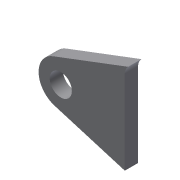
# Autodesk Inventor part: Soporte pivote freno
Saved by Autodesk Inventor 2019 (Build 230136000, 136)
## iProperties
Created: 2020-02-07
Part Number: Soporte pivote freno
Material: Generic
Document SubType Name: Modeling
Designer: Juan Carlos Botero
Density: 1 g/cm^3
Appearance: Default
Author: Juan Carlos Botero
Autodesk Inventor part; units mm, degrees
ref_plane "YZ Plane" through (0, 0, 0) normal (1, 0, 0) x (0, 1, 0)
ref_plane "XZ Plane" through (0, 0, 0) normal (0, 1, 0) x (-1, 0, 0)
ref_plane "XY Plane" through (0, 0, 0) normal (0, 0, 1) x (1, 0, 0)
sketch "Sketch1" plane through (0, 0, 0) normal (0, 0, 1) x (1, 0, 0)
  circle A0 centre (17.6912, 0) radius 5
  circle A1 centre (17.6912, 0) radius 10
  line L0 (17.2789, 9.9915) -> (48.052, 11.2613)
  ellipse E0 centre (55.5218, 7.7366) end of major axis (46.5416, 7.7366) minor radius 6.35 (55.5218, 14.0866) -> (46.5416, 7.7366) ccw
  line L1 (55.5218, 14.0866) -> (108.272, 14.0866)
  ellipse E1 centre (108.272, 7.7366) end of major axis (99.2917, 7.7366) minor radius 6.35 (117.2522, 7.7366) -> (108.272, 14.0866) ccw
  line L2 (117.2522, 7.7366) -> (117.2522, -29.5634)
  ellipse E2 centre (108.272, -29.5634) end of major axis (99.2917, -29.5634) minor radius 6.35 (108.272, -35.9134) -> (117.2522, -29.5634) ccw
  line L3 (108.272, -35.9134) -> (55.5218, -35.9134)
  ellipse E3 centre (55.5218, -29.5634) end of major axis (46.5416, -29.5634) minor radius 6.35 (46.5416, -29.5634) -> (55.5218, -35.9134) ccw
  line L4 (46.5416, -29.5634) -> (46.5416, 7.7366)
  line L5 (108.272, 10.9116) -> (55.5218, 10.9116)
  ellipse E4 centre (55.5218, 7.7366) end of major axis (51.0317, 7.7366) minor radius 3.175 (55.5218, 10.9116) -> (51.0317, 7.7366) ccw
  line L6 (51.0317, 7.7366) -> (51.0317, -29.5634)
  ellipse E5 centre (55.5218, -29.5634) end of major axis (51.0317, -29.5634) minor radius 3.175 (51.0317, -29.5634) -> (55.5218, -32.7384) ccw
  line L7 (55.5218, -32.7384) -> (108.272, -32.7384)
  ellipse E6 centre (108.272, -29.5634) end of major axis (103.7818, -29.5634) minor radius 3.175 (108.272, -32.7384) -> (112.7621, -29.5634) ccw
  line L8 (112.7621, -29.5634) -> (112.7621, 7.7366)
  ellipse E7 centre (108.272, 7.7366) end of major axis (103.7818, 7.7366) minor radius 3.175 (112.7621, 7.7366) -> (108.272, 10.9116) ccw
  circle A2 centre (-790.1228, -10.9134) radius 9.525 projected
  line L9 (46.5673, -30.0442) -> (12.355, -8.4572)
  dimension "d0" = 10
  dimension "d1" = 20
  constraints: 20 end point, 4 horizontal, 4 vertical, 2 centre point, 2 coincident, 2 point on circle, 2 tangent, 59 other
  measures "d0" diameter of A0
  measures "d1" diameter of A1
extrude "Extrusion1" add sketch "Sketch1" along normal blind 6 contours A1 | A1 L0 E0 L4 E3 L9
body "Solid1"
